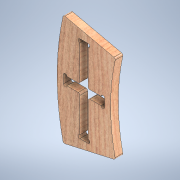
# Autodesk Inventor part: Feet
Saved by Autodesk Inventor 2021 (Build 250183000, 183)
## iProperties
Created: 2020-05-09
Part Number: Feet
Material: Wood (Birch)
Document SubType Name: Modeling
Designer: Dan Wikman
Density: 0.55 g/cm^3
Appearance: Birch - Natural Polished
Mass: 234.904 g
Surface Area: 715.223 cm^2
Volume: 427.099 cm^3
Autodesk Inventor part; units mm, degrees
ref_plane "YZ Plane" through (0, 0, 0) normal (1, 0, 0) x (0, 1, 0)
ref_plane "XZ Plane" through (0, 0, 0) normal (0, 1, 0) x (-1, 0, 0)
ref_plane "XY Plane" through (0, 0, 0) normal (0, 0, 1) x (1, 0, 0)
sketch "CONTOURS" plane through (0, 0, 0) normal (0, 0, 1) x (1, 0, 0)
  line L0 (2208.296, 893.1034) -> (2322.4299, 918.8568)
  arc A0 (2322.4299, 918.8568) -> (2325.4588, 923.6058) centre (2321.5495, 922.7587) ccw
  arc A1 (2325.4588, 1120.5613) -> (2325.4588, 923.6058) centre (2779.9113, 1022.0835) ccw
  arc A2 (2325.4588, 1120.5613) -> (2322.4299, 1125.3103) centre (2321.5495, 1121.4084) ccw
  line L1 (2322.4299, 1125.3103) -> (2208.296, 1151.0636)
  arc A3 (2208.296, 1151.0636) -> (2203.507, 1148.0122) centre (2207.4155, 1147.1617) ccw
  arc A4 (2203.507, 1148.0122) -> (2203.507, 896.1549) centre (2782.261, 1022.0835) ccw
  arc A5 (2203.507, 896.1549) -> (2208.296, 893.1034) centre (2207.4155, 897.0054) ccw
  constraints: 12 point on circle, 6 centre point, 4 end point
sketch "HOLES" plane through (0, 0, 0) normal (0, 0, 1) x (1, 0, 0)
  arc A0 (2243.3895, 1123.0835) -> (2243.3895, 1115.0835) centre (2243.3895, 1119.0835) ccw
  line L0 (2243.3895, 1115.0835) -> (2243.3895, 1035.5835)
  arc A1 (2239.3895, 1031.5835) -> (2243.3895, 1035.5835) centre (2239.3895, 1035.5835) ccw
  line L1 (2239.3895, 1031.5835) -> (2212.9126, 1031.5835)
  arc A2 (2212.9126, 1031.5835) -> (2204.9126, 1031.5835) centre (2208.9126, 1031.5835) ccw
  line L2 (2204.9126, 1031.5835) -> (2204.9126, 1012.5835)
  arc A3 (2204.9126, 1012.5835) -> (2212.9126, 1012.5835) centre (2208.9126, 1012.5835) ccw
  line L3 (2212.9126, 1012.5835) -> (2239.3895, 1012.5835)
  arc A4 (2243.3895, 1008.5835) -> (2239.3895, 1012.5835) centre (2239.3895, 1008.5835) ccw
  line L4 (2243.3895, 1008.5835) -> (2243.3895, 929.0835)
  arc A5 (2243.3895, 929.0835) -> (2243.3895, 921.0835) centre (2243.3895, 925.0835) ccw
  line L5 (2243.3895, 921.0835) -> (2262.3895, 921.0835)
  arc A6 (2262.3895, 921.0835) -> (2262.3895, 929.0835) centre (2262.3895, 925.0835) ccw
  line L6 (2262.3895, 929.0835) -> (2262.3895, 1008.5835)
  arc A7 (2266.3895, 1012.5835) -> (2262.3895, 1008.5835) centre (2266.3895, 1008.5835) ccw
  line L7 (2266.3895, 1012.5835) -> (2292.9126, 1012.5835)
  arc A8 (2292.9126, 1012.5835) -> (2300.9126, 1012.5835) centre (2296.9126, 1012.5835) ccw
  line L8 (2300.9126, 1012.5835) -> (2300.9126, 1031.5835)
  arc A9 (2300.9126, 1031.5835) -> (2292.9126, 1031.5835) centre (2296.9126, 1031.5835) ccw
  line L9 (2292.9126, 1031.5835) -> (2266.3895, 1031.5835)
  arc A10 (2262.3895, 1035.5835) -> (2266.3895, 1031.5835) centre (2266.3895, 1035.5835) ccw
  line L10 (2262.3895, 1035.5835) -> (2262.3895, 1115.0835)
  arc A11 (2262.3895, 1115.0835) -> (2262.3895, 1123.0835) centre (2262.3895, 1119.0835) ccw
  line L11 (2262.3895, 1123.0835) -> (2243.3895, 1123.0835)
  constraints: 24 end point, 24 point on circle, 12 centre point
extrude "Extrusion5" add sketch "CONTOURS" along normal blind 18
extrude "Extrusion6" cut sketch "HOLES" along normal blind 18
body "Solid1"
